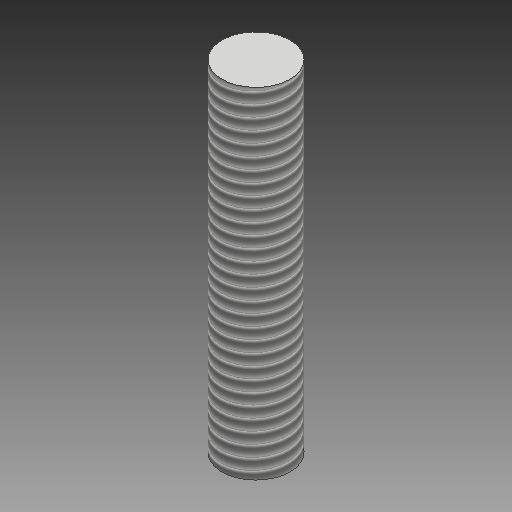
# Autodesk Inventor part: M5 Gewindestange
Saved by Autodesk Inventor 2019 (Build 230136000, 136)
## iProperties
Created: 2018-04-27
Part Number: M5 Gewindestange
Material: Generic
Document SubType Name: Modeling
Designer: Phil Erle
Density: 1 g/cm^3
Appearance: Default
Author: Phil Erle
Autodesk Inventor part; units mm, degrees
ref_plane "YZ Plane" through (0, 0, 0) normal (1, 0, 0) x (0, 1, 0)
ref_plane "XZ Plane" through (0, 0, 0) normal (0, 1, 0) x (-1, 0, 0)
ref_plane "XY Plane" through (0, 0, 0) normal (0, 0, 1) x (1, 0, 0)
sketch "Sketch1" plane through (0, 0, 0) normal (0, 0, 1) x (1, 0, 0)
  circle A0 centre (0, 0) radius 3
  dimension "d0" = 6
  constraints: 1 centre point, 1 coincident
  measures "d0" diameter of A0
extrude "Extrusion1" add sketch "Sketch1" along normal blind 30
thread "Thread1" size "M6x1" class "6g" standard "ISO Metric profile" full length
body "Solid1"
